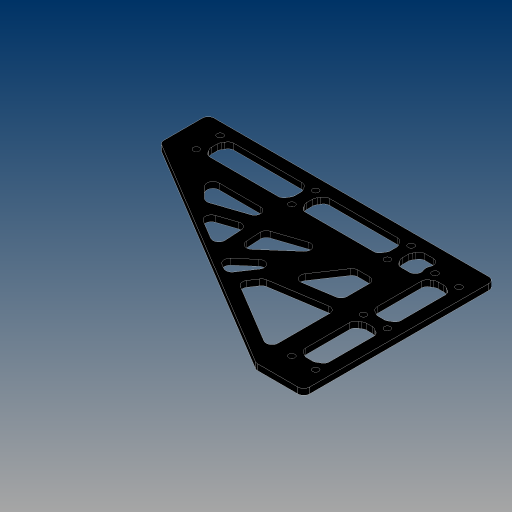
# Autodesk Inventor part: ELEV_042_ELEVTODRVBSE-MOUNT
Saved by Autodesk Inventor 2024.3 (Build 283343000, 343)
## iProperties
Created: 2024-12-07
Part Number: ELEV_042_ELEVTODRVBSE-MOUNT
Material: Steel
Document SubType Name: Modeling
Designer: Kenji
Mass: 1321.79 g
Surface Area: 708.184 cm^2
Volume: 168.38 cm^3
Density: 7.85 g/cm^3
Appearance: Anodized - Black
Author: Kenji
Autodesk Inventor part; units mm, degrees
ref_plane "YZ Plane" through (0, 0, 0) normal (1, 0, 0) x (0, 1, 0)
ref_plane "XZ Plane" through (0, 0, 0) normal (0, 1, 0) x (-1, 0, 0)
ref_plane "XY Plane" through (0, 0, 0) normal (0, 0, 1) x (1, 0, 0)
sketch "Sketch1" plane through (0, 0, 0) normal (0, 1, 0) x (-1, 0, 0)
  line L0 (0, 0) -> (254, 0) construction
  line L1 (254, 0) -> (254, -50.8) construction
  line L2 (254, -50.8) -> (0, -50.8) construction
  line L3 (0, -50.8) -> (0, 0) construction
  line L4 (0, 152.4) -> (-50.8, 152.4) construction
  line L5 (-50.8, 152.4) -> (-50.8, -50.8) construction
  line L6 (-50.8, -50.8) -> (0, -50.8) construction
  line L7 (0, -50.8) -> (0, 152.4) construction
  circle A0 centre (-12.7, 127) radius 3.2512
  circle A1 centre (-38.1, 127) radius 3.2512
  circle A2 centre (-12.7, 50.8) radius 3.2512
  circle A3 centre (-38.1, 50.8) radius 3.2512
  circle A4 centre (-12.7, -25.4) radius 3.2512
  circle A5 centre (-38.1, -25.4) radius 3.2512
  circle A6 centre (228.6, -12.7) radius 3.2512
  circle A7 centre (228.6, -38.1) radius 3.2512
  circle A8 centre (127, -12.7) radius 3.2512
  circle A9 centre (127, -38.1) radius 3.2512
  circle A10 centre (25.4, -12.7) radius 3.2512
  circle A11 centre (25.4, -38.1) radius 3.2512
  line L8 (254, -3.5953) -> (254, -44.45)
  line L9 (247.65, -50.8) -> (-44.45, -50.8)
  line L10 (-50.8, 146.05) -> (-50.8, -44.45)
  line L11 (1.5082, 151.4951) -> (250.917, 1.8498)
  line L12 (-1.7588, 152.4) -> (-44.45, 152.4)
  arc A12 (1.5082, 151.4951) -> (-1.7588, 152.4) centre (-1.7588, 146.05) ccw
  arc A13 (-44.45, 152.4) -> (-50.8, 146.05) centre (-44.45, 146.05) ccw
  arc A14 (-50.8, -44.45) -> (-44.45, -50.8) centre (-44.45, -44.45) ccw
  arc A15 (254, -3.5953) -> (250.917, 1.8498) centre (247.65, -3.5953) ccw
  arc A16 (247.65, -50.8) -> (254, -44.45) centre (247.65, -44.45) ccw
  dimension "d0" = 50.8
  dimension "d1" = 254
  dimension "d2" = 50.8
  dimension "d3" = 203.2
  dimension "d4" = 6.5024
  dimension "d5" = 25.4
  dimension "d8" = 12.7
  dimension "d9" = 25.4
  dimension "d12" = 76.2
  dimension "d17" = 12.7
  dimension "d18" = 25.4
  dimension "d19" = 6.5024
  dimension "d20" = 25.4
  dimension "d23" = 101.6
  dimension "d28" = 6.35
  constraints: 26 end point, 17 centre point, 10 point on circle, 10 point on line, 10 tangent, 6 equal radius, 4 collinear, 4 parallel, 4 perpendicular, 3 horizontal, 1 horizontal alignment, 1 vertical, 1 vertical alignment, 16 other
  measures "d0" distance between parallel lines of L2 L0
  measures "d1" distance between parallel lines of L3 L1
  measures "d2" distance between parallel lines of L5 L7
  measures "d3" distance between parallel lines of L6 L4
  measures "d4" diameter of A0
  measures "d5" distance from line of A0.centre L4
  measures "d8" distance from line of L7 A0.centre
  measures "d9" distance of A1.centre A0.centre
  measures "d12" distance of A0.centre A2.centre
  measures "d17" distance from line of L2 A7.centre
  measures "d18" distance of A6.centre A7.centre
  measures "d19" diameter of A7
  measures "d20" distance from line of L1 A6.centre
  measures "d23" distance of A6.centre A8.centre
  measures "d28" radius of A12
extrude "Extrusion1" add sketch "Sketch1" along normal blind 6.35
sketch "Sketch2" plane through (0, 6.35, 0) normal (0, 1, 0) x (1, 0, 0)
  line L0 (1.7588, -152.4) -> (44.45, -152.4) construction
  arc A0 (44.45, -152.4) -> (50.8, -146.05) centre (44.45, -146.05) ccw construction
  line L1 (50.8, -146.05) -> (50.8, 44.45) construction
  arc A1 (50.8, 44.45) -> (44.45, 50.8) centre (44.45, 44.45) ccw construction
  line L2 (44.45, 50.8) -> (-247.65, 50.8) construction
  arc A2 (-247.65, 50.8) -> (-254, 44.45) centre (-247.65, 44.45) ccw construction
  line L3 (-254, 44.45) -> (-254, 3.5953) construction
  arc A3 (-254, 3.5953) -> (-250.917, -1.8498) centre (-247.65, 3.5953) ccw construction
  line L4 (-250.917, -1.8498) -> (-1.5082, -151.4951) construction
  arc A4 (-1.5082, -151.4951) -> (1.7588, -152.4) centre (1.7588, -146.05) ccw construction
  circle A5 centre (-25.4, 38.1) radius 3.2512 construction
  circle A6 centre (-127, 38.1) radius 3.2512 construction
  circle A7 centre (-228.6, 38.1) radius 3.2512 construction
  circle A8 centre (-228.6, 12.7) radius 3.2512 construction
  circle A9 centre (38.1, 25.4) radius 3.2512 construction
  circle A10 centre (12.7, 25.4) radius 3.2512 construction
  circle A11 centre (38.1, -50.8) radius 3.2512 construction
  circle A12 centre (12.7, -50.8) radius 3.2512 construction
  circle A13 centre (38.1, -127) radius 3.2512 construction
  circle A14 centre (12.7, -127) radius 3.2512 construction
  circle A15 centre (-127, 12.7) radius 3.2512 construction
  circle A16 centre (-25.4, 12.7) radius 3.2512 construction
  line L5 (1.7588, -146.05) -> (-247.65, 3.5953) construction
  line L6 (-247.65, 3.5953) -> (-247.65, 44.45) construction
  line L7 (-247.65, 44.45) -> (44.45, 44.45) construction
  line L8 (44.45, 44.45) -> (44.45, -146.05) construction
  line L9 (44.45, -146.05) -> (1.7588, -146.05) construction
  circle A17 centre (-228.6, 12.7) radius 9.6012 construction
  circle A18 centre (-228.6, 38.1) radius 9.6012 construction
  circle A19 centre (-127, 12.7) radius 9.6012 construction
  circle A20 centre (-127, 38.1) radius 9.6012 construction
  circle A21 centre (-25.4, 12.7) radius 9.6012 construction
  circle A22 centre (-25.4, 38.1) radius 9.6012 construction
  circle A23 centre (12.7, 25.4) radius 9.6012 construction
  circle A24 centre (38.1, 25.4) radius 9.6012 construction
  circle A25 centre (12.7, -50.8) radius 9.6012 construction
  circle A26 centre (38.1, -50.8) radius 9.6012 construction
  circle A27 centre (12.7, -127) radius 9.6012 construction
  circle A28 centre (38.1, -127) radius 9.6012 construction
  line L10 (0, 0) -> (0, -152.1516) construction
  line L11 (6.35, 0) -> (6.35, -146.05) construction
  line L12 (-6.35, 0) -> (-6.35, -141.1847) construction
  line L13 (0, 0) -> (-254, 0) construction
  line L14 (0, 6.35) -> (-247.65, 6.35) construction
  line L15 (-6.35, -6.35) -> (-231.0745, -6.35) construction
  line L16 (12.7, -50.8) -> (-93.4912, -88.9) construction
  line L17 (12.7, -127) -> (-93.4912, -88.9) construction
  line L18 (-25.4, 12.7) -> (-93.4912, -88.9) construction
  line L19 (-25.4, 12.7) -> (-177.8, -38.3147) construction
  line L20 (-127, 12.7) -> (-177.8, -38.3147) construction
  line L21 (-228.6, 12.7) -> (-177.8, -38.3147) construction
  line L22 (-127, 12.7) -> (-122.0107, -71.7883) construction
  line L23 (-122.0107, -71.7883) -> (12.7, -50.8) construction
  line L24 (-25.4, 12.7) -> (-122.0107, -71.7883) construction
  line L25 (-36.6651, -15.5148) -> (-55.9466, -44.2851)
  line L26 (-49.6941, -54.0946) -> (-18.0724, -49.1678)
  line L27 (-12.7, -19.05) -> (-12.7, -42.8935)
  line L28 (-19.05, -12.7) -> (-31.3901, -12.7)
  arc A29 (-55.9466, -44.2851) -> (-49.6941, -54.0946) centre (-50.6716, -47.8203) ccw
  arc A30 (-31.3901, -12.7) -> (-36.6651, -15.5148) centre (-31.3901, -19.05) ccw
  arc A31 (-12.7, -19.05) -> (-19.05, -12.7) centre (-19.05, -19.05) ccw
  arc A32 (-18.0724, -49.1678) -> (-12.7, -42.8935) centre (-19.05, -42.8935) ccw
  line L29 (-118.1184, -29.9818) -> (-117.1996, -45.5403)
  line L30 (-83.4828, -13.4391) -> (-113.7951, -23.5859)
  line L31 (-77.2869, -24.2407) -> (-106.6805, -49.946)
  arc A33 (-117.1996, -45.5403) -> (-106.6805, -49.946) centre (-110.8607, -45.166) ccw
  arc A34 (-113.7951, -23.5859) -> (-118.1184, -29.9818) centre (-111.7795, -29.6075) ccw
  arc A35 (-77.2869, -24.2407) -> (-83.4828, -13.4391) centre (-81.4672, -19.4607) ccw
  line L32 (-93.835, -55.5838) -> (-109.7268, -69.4814)
  line L33 (-84.3799, -63.8989) -> (-95.5804, -80.6114)
  arc A36 (-84.3799, -63.8989) -> (-93.835, -55.5838) centre (-89.6548, -60.3637) ccw
  line L34 (-104.1224, -82.5213) -> (-108.8136, -79.7065)
  arc A37 (-109.7268, -69.4814) -> (-108.8136, -79.7065) centre (-105.5466, -74.2614) ccw
  arc A38 (-104.1224, -82.5213) -> (-95.5804, -80.6114) centre (-100.8553, -77.0762) ccw
  line L35 (-138.7462, -31.9381) -> (-157.5657, -38.2378)
  line L36 (-130.3915, -37.5853) -> (-129.3145, -55.823)
  line L37 (-158.8171, -49.7044) -> (-138.9205, -61.6424)
  arc A39 (-157.5657, -38.2378) -> (-158.8171, -49.7044) centre (-155.5501, -44.2593) ccw
  arc A40 (-130.3915, -37.5853) -> (-138.7462, -31.9381) centre (-136.7305, -37.9596) ccw
  arc A41 (-138.9205, -61.6424) -> (-129.3145, -55.823) centre (-135.6535, -56.1973) ccw
  line L38 (-189.8837, -17.1807) -> (-178.8597, -28.2512)
  line L39 (-139.2725, -18.7216) -> (-172.3445, -29.7922)
  line L40 (-132.2361, -6.35) -> (-131.6561, -16.1721)
  line L41 (-185.3841, -6.35) -> (-141.2882, -6.35)
  arc A42 (-185.3841, -6.35) -> (-189.8837, -17.1807) centre (-185.3841, -12.7) ccw
  arc A43 (-178.8597, -28.2512) -> (-172.3445, -29.7922) centre (-174.3601, -23.7706) ccw
  arc A44 (-139.2725, -18.7216) -> (-141.2882, -6.35) centre (-141.2882, -12.7) ccw
  line L42 (-75.1834, -72.9886) -> (-80.783, -81.344)
  line L43 (-70.886, -70.2495) -> (-13.6776, -61.3363)
  line L44 (-6.35, -67.6106) -> (-6.35, -122.5641)
  arc A45 (-6.35, -67.6106) -> (-13.6776, -61.3363) centre (-12.7, -67.6106) ccw
  arc A46 (-70.886, -70.2495) -> (-75.1834, -72.9886) centre (-69.9084, -76.5238) ccw
  line L45 (-15.967, -128.0092) -> (-78.7752, -90.3243)
  arc A47 (-80.783, -81.344) -> (-78.7752, -90.3243) centre (-75.5081, -84.8792) ccw
  arc A48 (-15.967, -128.0092) -> (-6.35, -122.5641) centre (-12.7, -122.5641) ccw
  point P0 (-116.2897, -75.2209)
  point P1 (-98.9431, -85.6289)
  point P2 (-170.6362, -42.613)
  point P3 (-128.6054, -67.8315)
  point P4 (-200.6688, -6.35)
  point P5 (-6.35, -60.1947)
  dimension "d34" = 6.35
  dimension "d35" = 6.35
  dimension "d36" = 6.35
  dimension "d37" = 6.35
  dimension "d38" = 6.35
  dimension "d39" = 6.35
  dimension "d40" = 6.35
  dimension "d41" = 6.35
  dimension "d42" = 6.35
  dimension "d43" = 6.35
  dimension "d44" = 6.35
  dimension "d45" = 6.35
  dimension "d46" = 6.35
  dimension "d47" = 6.35
  dimension "d48" = 6.35
  dimension "d49" = 6.35
  dimension "d50" = 6.35
  dimension "d57" = 15
  dimension "d62" = 6.35
  dimension "d63" = 6.35
  dimension "d64" = 6.35
  dimension "d65" = 6.35
  dimension "d66" = 6.35
  dimension "d67" = 6.35
  dimension "d68" = 6.35
  dimension "d69" = 6.35
  dimension "d70" = 6.35
  dimension "d71" = 6.35
  dimension "d72" = 6.35
  dimension "d73" = 6.35
  dimension "d74" = 6.35
  dimension "d75" = 6.35
  dimension "d76" = 6.35
  dimension "d77" = 6.35
  dimension "d78" = 6.35
  dimension "d79" = 6.35
  dimension "d80" = 6.35
  dimension "d81" = 6.35
  dimension "d82" = 6.35
  dimension "d83" = 6.35
  dimension "d84" = 6.35
  dimension "d90" = 6.35
  dimension "d91" = 6.35
  dimension "d92" = 6.35
  constraints: 80 end point, 41 point on circle, 40 tangent, 32 centre point, 22 point on line, 20 parallel, 11 equal radius, 2 collinear, 2 equal length, 2 horizontal alignment, 1 horizontal, 1 vertical, 19 other
  measures "d35" radial gap between concentric circles of A8 A17
  measures "d36" radial gap between concentric circles of A7 A18
  measures "d37" radial gap between concentric circles of A15 A19
  measures "d38" radial gap between concentric circles of A6 A20
  measures "d39" radial gap between concentric circles of A16 A21
  measures "d40" radial gap between concentric circles of A5 A22
  measures "d41" radial gap between concentric circles of A10 A23
  measures "d42" radial gap between concentric circles of A9 A24
  measures "d43" radial gap between concentric circles of A12 A25
  measures "d44" radial gap between concentric circles of A11 A26
  measures "d45" radial gap between concentric circles of A14 A27
  measures "d46" radial gap between concentric circles of A13 A28
  measures "d47" distance between parallel lines of L10 L11
  measures "d48" distance between parallel lines of L10 L12
  measures "d49" distance between parallel lines of L13 L14
  measures "d50" distance between parallel lines of L13 L15
  measures "d57" angle of L18 L24
  measures "d62" distance between parallel lines of L18 L25
  measures "d63" distance between parallel lines of L23 L26
  measures "d64" distance between parallel lines of L12 L27
  measures "d65" distance between parallel lines of L15 L28
  measures "d66" radius of A29
  measures "d67" distance between parallel lines of L22 L29
  measures "d68" distance between parallel lines of L19 L30
  measures "d69" distance between parallel lines of L24 L31
  measures "d70" radius of A33
  measures "d71" distance between parallel lines of L24 L32
  measures "d72" distance between parallel lines of L18 L33
  measures "d73" radius of A36
  measures "d74" radius of A37
  measures "d75" distance between parallel lines of L19 L35
  measures "d76" distance between parallel lines of L22 L36
  measures "d77" radius of A39
  measures "d78" distance between parallel lines of L21 L38
  measures "d79" distance between parallel lines of L19 L39
  measures "d80" distance between parallel lines of L22 L40
  measures "d81" radius of A42
  measures "d82" radius of A43
  measures "d83" distance between parallel lines of L18 L42
  measures "d84" distance between parallel lines of L23 L43
  measures "d90" radius of A45
  measures "d92" radius of A47
extrude "Extrusion3" cut sketch "Sketch2" against normal blind 6.35
sketch "Sketch3" plane through (0, 6.35, 0) normal (0, 1, 0) x (1, 0, 0)
  arc A0 (-113.7951, -23.5859) -> (-118.1184, -29.9818) centre (-111.7795, -29.6075) ccw construction
  line L0 (-113.7951, -23.5859) -> (-83.4828, -13.4391) construction
  arc A1 (-77.2869, -24.2407) -> (-83.4828, -13.4391) centre (-81.4672, -19.4607) ccw construction
  line L1 (-77.2869, -24.2407) -> (-106.6805, -49.946) construction
  arc A2 (-117.1996, -45.5403) -> (-106.6805, -49.946) centre (-110.8607, -45.166) ccw construction
  line L2 (-117.1996, -45.5403) -> (-118.1184, -29.9818) construction
  arc A3 (-31.3901, -12.7) -> (-36.6651, -15.5148) centre (-31.3901, -19.05) ccw construction
  line L3 (-31.3901, -12.7) -> (-19.05, -12.7) construction
  arc A4 (-12.7, -19.05) -> (-19.05, -12.7) centre (-19.05, -19.05) ccw construction
  line L4 (-12.7, -19.05) -> (-12.7, -42.8935) construction
  arc A5 (-18.0724, -49.1678) -> (-12.7, -42.8935) centre (-19.05, -42.8935) ccw construction
  line L5 (-18.0724, -49.1678) -> (-49.6941, -54.0946) construction
  arc A6 (-55.9466, -44.2851) -> (-49.6941, -54.0946) centre (-50.6716, -47.8203) ccw construction
  line L6 (-55.9466, -44.2851) -> (-36.6651, -15.5148) construction
  arc A7 (-157.5657, -38.2378) -> (-158.8171, -49.7044) centre (-155.5501, -44.2593) ccw construction
  line L7 (-157.5657, -38.2378) -> (-138.7462, -31.9381) construction
  arc A8 (-130.3915, -37.5853) -> (-138.7462, -31.9381) centre (-136.7305, -37.9596) ccw construction
  line L8 (-130.3915, -37.5853) -> (-129.3145, -55.823) construction
  arc A9 (-138.9205, -61.6424) -> (-129.3145, -55.823) centre (-135.6535, -56.1973) ccw construction
  line L9 (-138.9205, -61.6424) -> (-158.8171, -49.7044) construction
  arc A10 (-109.7268, -69.4814) -> (-108.8136, -79.7065) centre (-105.5466, -74.2614) ccw construction
  line L10 (-109.7268, -69.4814) -> (-93.835, -55.5838) construction
  arc A11 (-84.3799, -63.8989) -> (-93.835, -55.5838) centre (-89.6548, -60.3637) ccw construction
  line L11 (-84.3799, -63.8989) -> (-95.5804, -80.6114) construction
  arc A12 (-104.1224, -82.5213) -> (-95.5804, -80.6114) centre (-100.8553, -77.0762) ccw construction
  line L12 (-104.1224, -82.5213) -> (-108.8136, -79.7065) construction
  arc A13 (-80.783, -81.344) -> (-78.7752, -90.3243) centre (-75.5081, -84.8792) ccw construction
  line L13 (-80.783, -81.344) -> (-75.1834, -72.9886) construction
  arc A14 (-70.886, -70.2495) -> (-75.1834, -72.9886) centre (-69.9084, -76.5238) ccw construction
  line L14 (-70.886, -70.2495) -> (-13.6776, -61.3363) construction
  arc A15 (-6.35, -67.6106) -> (-13.6776, -61.3363) centre (-12.7, -67.6106) ccw construction
  line L15 (-6.35, -67.6106) -> (-6.35, -122.5641) construction
  arc A16 (-15.967, -128.0092) -> (-6.35, -122.5641) centre (-12.7, -122.5641) ccw construction
  line L16 (-15.967, -128.0092) -> (-78.7752, -90.3243) construction
  arc A17 (-178.8597, -28.2512) -> (-172.3445, -29.7922) centre (-174.3601, -23.7706) ccw construction
  line L17 (-178.8597, -28.2512) -> (-189.8837, -17.1807) construction
  arc A18 (-185.3841, -6.35) -> (-189.8837, -17.1807) centre (-185.3841, -12.7) ccw construction
  line L18 (-185.3841, -6.35) -> (-141.2882, -6.35) construction
  arc A19 (-139.2725, -18.7216) -> (-141.2882, -6.35) centre (-141.2882, -12.7) ccw construction
  line L19 (-139.2725, -18.7216) -> (-172.3445, -29.7922) construction
  line L20 (1.7588, -152.4) -> (44.45, -152.4) construction
  arc A20 (44.45, -152.4) -> (50.8, -146.05) centre (44.45, -146.05) ccw construction
  line L21 (50.8, -146.05) -> (50.8, 44.45) construction
  arc A21 (50.8, 44.45) -> (44.45, 50.8) centre (44.45, 44.45) ccw construction
  line L22 (44.45, 50.8) -> (-247.65, 50.8) construction
  arc A22 (-247.65, 50.8) -> (-254, 44.45) centre (-247.65, 44.45) ccw construction
  line L23 (-254, 44.45) -> (-254, 3.5953) construction
  arc A23 (-254, 3.5953) -> (-250.917, -1.8498) centre (-247.65, 3.5953) ccw construction
  line L24 (-250.917, -1.8498) -> (-1.5082, -151.4951) construction
  arc A24 (-1.5082, -151.4951) -> (1.7588, -152.4) centre (1.7588, -146.05) ccw construction
  circle A25 centre (-25.4, 38.1) radius 3.2512 construction
  circle A26 centre (-127, 38.1) radius 3.2512 construction
  circle A27 centre (-228.6, 38.1) radius 3.2512 construction
  circle A28 centre (-228.6, 12.7) radius 3.2512 construction
  circle A29 centre (38.1, 25.4) radius 3.2512 construction
  circle A30 centre (12.7, 25.4) radius 3.2512 construction
  circle A31 centre (38.1, -50.8) radius 3.2512 construction
  circle A32 centre (12.7, -50.8) radius 3.2512 construction
  circle A33 centre (38.1, -127) radius 3.2512 construction
  circle A34 centre (12.7, -127) radius 3.2512 construction
  circle A35 centre (-127, 12.7) radius 3.2512 construction
  circle A36 centre (-25.4, 12.7) radius 3.2512 construction
  line L25 (-252.8841, 0) -> (0, 0) construction
  line L26 (0, 0) -> (0, -152.1516) construction
  line L27 (-247.65, 6.35) -> (-247.65, 44.45) construction
  line L28 (-247.65, 44.45) -> (44.45, 44.45) construction
  line L29 (44.45, 44.45) -> (44.45, -146.05) construction
  line L30 (44.45, -146.05) -> (6.35, -146.05) construction
  line L31 (6.35, 6.35) -> (6.35, -146.05) construction
  line L32 (-247.65, 6.35) -> (6.35, 6.35) construction
  circle A37 centre (12.7, -127) radius 9.6012 construction
  circle A38 centre (38.1, -127) radius 9.6012 construction
  circle A39 centre (12.7, -50.8) radius 9.6012 construction
  circle A40 centre (38.1, -50.8) radius 9.6012 construction
  circle A41 centre (12.7, 25.4) radius 9.6012 construction
  circle A42 centre (38.1, 25.4) radius 9.6012 construction
  circle A43 centre (-25.4, 12.7) radius 9.6012 construction
  circle A44 centre (-25.4, 38.1) radius 9.6012 construction
  circle A45 centre (-127, 12.7) radius 9.6012 construction
  circle A46 centre (-127, 38.1) radius 9.6012 construction
  circle A47 centre (-228.6, 12.7) radius 9.6012 construction
  circle A48 centre (-228.6, 38.1) radius 9.6012 construction
  line L33 (-228.6, 22.3012) -> (-228.6, 28.4988) construction
  line L34 (-127, 22.3012) -> (-127, 28.4988) construction
  line L35 (-222.25, 22.3515) -> (-222.25, 28.4485)
  line L36 (-213.9672, 38.1) -> (-141.6328, 38.1)
  line L37 (-213.9672, 12.7) -> (-141.6328, 12.7)
  line L38 (-133.35, 22.3515) -> (-133.35, 28.4485)
  arc A49 (-134.6443, 18.5093) -> (-135.8076, 16.5221) centre (-127, 12.7) ccw
  arc A50 (-135.8076, 34.2779) -> (-134.6443, 32.2907) centre (-127, 38.1) ccw
  arc A51 (-219.7924, 16.5221) -> (-220.9557, 18.5093) centre (-228.6, 12.7) ccw
  arc A52 (-220.9557, 32.2907) -> (-219.7924, 34.2779) centre (-228.6, 38.1) ccw
  arc A53 (-222.25, 22.3515) -> (-220.9557, 18.5093) centre (-215.9, 22.3515) ccw
  arc A54 (-220.9557, 32.2907) -> (-222.25, 28.4485) centre (-215.9, 28.4485) ccw
  arc A55 (-213.9672, 38.1) -> (-219.7924, 34.2779) centre (-213.9672, 31.75) ccw
  arc A56 (-219.7924, 16.5221) -> (-213.9672, 12.7) centre (-213.9672, 19.05) ccw
  arc A57 (-141.6328, 12.7) -> (-135.8076, 16.5221) centre (-141.6328, 19.05) ccw
  arc A58 (-134.6443, 18.5093) -> (-133.35, 22.3515) centre (-139.7, 22.3515) ccw
  arc A59 (-133.35, 28.4485) -> (-134.6443, 32.2907) centre (-139.7, 28.4485) ccw
  arc A60 (-135.8076, 34.2779) -> (-141.6328, 38.1) centre (-141.6328, 31.75) ccw
  line L39 (-120.65, 22.3515) -> (-120.65, 28.4485)
  line L40 (-112.3672, 12.7) -> (-40.0328, 12.7)
  line L41 (-112.3672, 38.1) -> (-40.0328, 38.1)
  line L42 (-25.4, 28.4988) -> (-25.4, 22.3012) construction
  arc A61 (-119.3557, 32.2907) -> (-118.1924, 34.2779) centre (-127, 38.1) ccw
  arc A62 (-118.1924, 16.5221) -> (-119.3557, 18.5093) centre (-127, 12.7) ccw
  line L43 (-31.75, 28.4485) -> (-31.75, 22.3515)
  arc A63 (-33.0443, 18.5093) -> (-34.2076, 16.5221) centre (-25.4, 12.7) ccw
  arc A64 (-34.2076, 34.2779) -> (-33.0443, 32.2907) centre (-25.4, 38.1) ccw
  arc A65 (-33.0443, 18.5093) -> (-31.75, 22.3515) centre (-38.1, 22.3515) ccw
  arc A66 (-31.75, 28.4485) -> (-33.0443, 32.2907) centre (-38.1, 28.4485) ccw
  arc A67 (-34.2076, 34.2779) -> (-40.0328, 38.1) centre (-40.0328, 31.75) ccw
  arc A68 (-40.0328, 12.7) -> (-34.2076, 16.5221) centre (-40.0328, 19.05) ccw
  arc A69 (-118.1924, 16.5221) -> (-112.3672, 12.7) centre (-112.3672, 19.05) ccw
  arc A70 (-120.65, 22.3515) -> (-119.3557, 18.5093) centre (-114.3, 22.3515) ccw
  arc A71 (-119.3557, 32.2907) -> (-120.65, 28.4485) centre (-114.3, 28.4485) ccw
  arc A72 (-112.3672, 38.1) -> (-118.1924, 34.2779) centre (-112.3672, 31.75) ccw
  line L44 (22.3012, -50.8) -> (28.4988, -50.8) construction
  line L45 (22.3012, -127) -> (28.4988, -127) construction
  line L46 (22.3012, 25.4) -> (28.4988, 25.4) construction
  line L47 (12.7, -65.4328) -> (12.7, -112.3672)
  line L48 (38.1, -65.4328) -> (38.1, -112.3672)
  line L49 (22.3515, -120.65) -> (28.4485, -120.65)
  line L50 (22.3515, -57.15) -> (28.4485, -57.15)
  arc A73 (18.5093, -119.3557) -> (16.5221, -118.1924) centre (12.7, -127) ccw
  arc A74 (34.2779, -118.1924) -> (32.2907, -119.3557) centre (38.1, -127) ccw
  arc A75 (16.5221, -59.6076) -> (18.5093, -58.4443) centre (12.7, -50.8) ccw
  arc A76 (32.2907, -58.4443) -> (34.2779, -59.6076) centre (38.1, -50.8) ccw
  arc A77 (18.5093, -119.3557) -> (22.3515, -120.65) centre (22.3515, -114.3) ccw
  arc A78 (12.7, -112.3672) -> (16.5221, -118.1924) centre (19.05, -112.3672) ccw
  arc A79 (28.4485, -120.65) -> (32.2907, -119.3557) centre (28.4485, -114.3) ccw
  arc A80 (34.2779, -118.1924) -> (38.1, -112.3672) centre (31.75, -112.3672) ccw
  arc A81 (38.1, -65.4328) -> (34.2779, -59.6076) centre (31.75, -65.4328) ccw
  arc A82 (32.2907, -58.4443) -> (28.4485, -57.15) centre (28.4485, -63.5) ccw
  arc A83 (22.3515, -57.15) -> (18.5093, -58.4443) centre (22.3515, -63.5) ccw
  arc A84 (16.5221, -59.6076) -> (12.7, -65.4328) centre (19.05, -65.4328) ccw
  line L51 (22.3515, -44.45) -> (28.4485, -44.45)
  line L52 (22.3515, 19.05) -> (28.4485, 19.05)
  line L53 (12.7, 10.7672) -> (12.7, -36.1672)
  line L54 (38.1, 10.7672) -> (38.1, -36.1672)
  arc A85 (18.5093, -43.1557) -> (16.5221, -41.9924) centre (12.7, -50.8) ccw
  arc A86 (34.2779, -41.9924) -> (32.2907, -43.1557) centre (38.1, -50.8) ccw
  arc A87 (16.5221, 16.5924) -> (18.5093, 17.7557) centre (12.7, 25.4) ccw
  arc A88 (32.2907, 17.7557) -> (34.2779, 16.5924) centre (38.1, 25.4) ccw
  arc A89 (16.5221, 16.5924) -> (12.7, 10.7672) centre (19.05, 10.7672) ccw
  arc A90 (22.3515, 19.05) -> (18.5093, 17.7557) centre (22.3515, 12.7) ccw
  arc A91 (32.2907, 17.7557) -> (28.4485, 19.05) centre (28.4485, 12.7) ccw
  arc A92 (38.1, 10.7672) -> (34.2779, 16.5924) centre (31.75, 10.7672) ccw
  arc A93 (34.2779, -41.9924) -> (38.1, -36.1672) centre (31.75, -36.1672) ccw
  arc A94 (18.5093, -43.1557) -> (22.3515, -44.45) centre (22.3515, -38.1) ccw
  arc A95 (28.4485, -44.45) -> (32.2907, -43.1557) centre (28.4485, -38.1) ccw
  arc A96 (12.7, -36.1672) -> (16.5221, -41.9924) centre (19.05, -36.1672) ccw
  line L55 (12.7, 25.4) -> (12.7, 35.0012) construction
  line L56 (-19.05, 28.4485) -> (-19.05, 22.3515)
  line L57 (-10.7672, 12.7) -> (-1.9328, 12.7)
  line L58 (-10.7672, 38.1) -> (-1.9328, 38.1)
  arc A97 (3.8924, 29.2221) -> (3.8924, 21.5779) centre (12.7, 25.4) ccw
  arc A98 (-16.5924, 16.5221) -> (-17.7557, 18.5093) centre (-25.4, 12.7) ccw
  arc A99 (-17.7557, 32.2907) -> (-16.5924, 34.2779) centre (-25.4, 38.1) ccw
  arc A100 (-19.05, 22.3515) -> (-17.7557, 18.5093) centre (-12.7, 22.3515) ccw
  arc A101 (-16.5924, 16.5221) -> (-10.7672, 12.7) centre (-10.7672, 19.05) ccw
  arc A102 (-17.7557, 32.2907) -> (-19.05, 28.4485) centre (-12.7, 28.4485) ccw
  arc A103 (-10.7672, 38.1) -> (-16.5924, 34.2779) centre (-10.7672, 31.75) ccw
  circle A104 centre (-1.9328, 31.75) radius 6.35 construction
  arc A105 (3.8924, 29.2221) -> (-1.9328, 38.1) centre (-1.9328, 31.75) ccw
  circle A106 centre (-1.9328, 19.05) radius 6.35 construction
  arc A107 (-1.9328, 12.7) -> (3.8924, 21.5779) centre (-1.9328, 19.05) ccw
  point P0 (-222.25, 19.9014)
  point P1 (-222.25, 30.8986)
  point P2 (-218.9988, 38.1)
  point P3 (-136.6012, 38.1)
  point P4 (-136.6012, 12.7)
  point P5 (-133.35, 19.9014)
  point P6 (-133.35, 30.8986)
  point P7 (-218.9988, 12.7)
  point P8 (-120.65, 19.9014)
  point P9 (-120.65, 30.8986)
  point P10 (-117.3988, 12.7)
  point P11 (-35.0012, 12.7)
  point P12 (-117.3988, 38.1)
  point P13 (-35.0012, 38.1)
  point P14 (-31.75, 30.8986)
  point P15 (-31.75, 19.9014)
  point P16 (12.7, -60.4012)
  point P17 (12.7, -117.3988)
  point P18 (38.1, -60.4012)
  point P19 (38.1, -117.3988)
  point P20 (19.9014, -120.65)
  point P21 (30.8986, -120.65)
  point P22 (19.9014, -57.15)
  point P23 (30.8986, -57.15)
  point P24 (38.1, -117.3988)
  point P25 (19.9014, -44.45)
  point P26 (30.8986, -44.45)
  point P27 (19.9014, 19.05)
  point P28 (30.8986, 19.05)
  point P29 (12.7, 15.7988)
  point P30 (12.7, -41.1988)
  point P31 (38.1, 15.7988)
  point P32 (38.1, -41.1988)
  point P33 (-19.05, 30.8986)
  point P34 (-19.05, 19.9014)
  point P35 (-15.7988, 12.7)
  point P36 (-15.7988, 38.1)
  dimension "d95" = 6.35
  dimension "d96" = 6.35
  dimension "d97" = 6.35
  dimension "d98" = 6.35
  dimension "d99" = 6.35
  dimension "d100" = 6.35
  dimension "d101" = 6.35
  dimension "d102" = 6.35
  dimension "d103" = 6.35
  dimension "d104" = 6.35
  dimension "d105" = 6.35
  dimension "d106" = 6.35
  dimension "d107" = 6.35
  dimension "d108" = 6.35
  dimension "d109" = 6.35
  dimension "d110" = 6.35
  dimension "d111" = 6.35
  dimension "d112" = 6.35
  dimension "d113" = 6.35
  dimension "d114" = 6.35
  dimension "d115" = 6.35
  dimension "d116" = 6.35
  dimension "d117" = 6.35
  dimension "d118" = 6.35
  dimension "d119" = 6.35
  dimension "d120" = 6.35
  dimension "d121" = 6.35
  dimension "d122" = 6.35
  dimension "d123" = 6.35
  dimension "d124" = 6.35
  dimension "d125" = 6.35
  dimension "d126" = 6.35
  dimension "d127" = 6.35
  dimension "d128" = 6.35
  dimension "d129" = 6.35
  dimension "d135" = 6.35
  dimension "d136" = 6.35
  dimension "d137" = 6.35
  dimension "d138" = 6.35
  dimension "d139" = 12.7
  dimension "d140" = 12.7
  constraints: 207 point on circle, 78 tangent, 71 centre point, 68 end point, 50 equal radius, 47 point on line, 24 parallel, 3 horizontal, 3 vertical, 2 concentric, 1 perpendicular, 3 other
  measures "d95" distance between parallel lines of L23 L27
  measures "d96" distance between parallel lines of L26 L31
  measures "d97" distance between parallel lines of L25 L32
  measures "d98" radial gap between concentric circles of A34 A37
  measures "d99" radial gap between concentric circles of A33 A38
  measures "d100" radial gap between concentric circles of A32 A39
  measures "d101" radial gap between concentric circles of A31 A40
  measures "d102" radial gap between concentric circles of A30 A41
  measures "d103" radial gap between concentric circles of A29 A42
  measures "d104" radial gap between concentric circles of A36 A43
  measures "d105" radial gap between concentric circles of A25 A44
  measures "d106" radial gap between concentric circles of A35 A45
  measures "d107" radial gap between concentric circles of A26 A46
  measures "d108" radial gap between concentric circles of A28 A47
  measures "d109" radial gap between concentric circles of A27 A48
  measures "d110" distance between parallel lines of L33 L35
  measures "d111" distance between parallel lines of L28 L36
  measures "d112" distance between parallel lines of L32 L37
  measures "d113" distance between parallel lines of L34 L38
  measures "d114" radius of A53
  measures "d115" distance between parallel lines of L34 L39
  measures "d116" distance between parallel lines of L32 L40
  measures "d117" distance between parallel lines of L28 L41
  measures "d118" distance between parallel lines of L42 L43
  measures "d119" radius of A65
  measures "d120" distance between parallel lines of L31 L47
  measures "d121" distance between parallel lines of L29 L48
  measures "d122" distance between parallel lines of L45 L49
  measures "d123" distance between parallel lines of L44 L50
  measures "d124" radius of A77
  measures "d125" distance between parallel lines of L44 L51
  measures "d126" distance between parallel lines of L46 L52
  measures "d127" distance between parallel lines of L31 L53
  measures "d128" distance between parallel lines of L29 L54
  measures "d129" radius of A89
  measures "d135" distance between parallel lines of L42 L56
  measures "d136" distance between parallel lines of L32 L57
  measures "d137" distance between parallel lines of L28 L58
  measures "d138" radius of A100
  measures "d139" diameter of A104
  measures "d140" diameter of A106
extrude "Extrusion4" cut sketch "Sketch3" against normal blind 6.35
body "Solid1"
